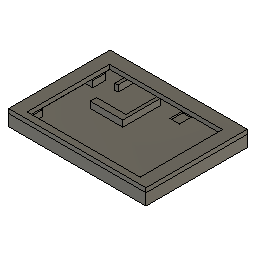
tty-buddy-enclosure (Autodesk Fusion 360 design; units mm, degrees)
part number: 2026-09-05-10-40-58-027
Autodesk Fusion 360 part; units mm, degrees
sketch "body_base" plane through (0, 0, 0) normal (0, 0, 1) x (1, 0, 0)
  line L0 (40.5, -27.25) -> (-40.5, -27.25)
  line L1 (-40.5, -27.25) -> (-40.5, 27.25)
  line L2 (-40.5, 27.25) -> (40.5, 27.25)
  line L3 (40.5, 27.25) -> (40.5, -27.25)
  line L4 (40.5, -27.25) -> (-40.5, 27.25) construction
  line L5 (-40.5, -27.25) -> (40.5, 27.25) construction
  line L6 (-40.5, 27.25) -> (40.5, 27.25)
  line L7 (40.5, 27.25) -> (40.5, 31.25)
  line L8 (40.5, 31.25) -> (-40.5, 31.25)
  line L9 (-40.5, 31.25) -> (-40.5, 27.25)
  line L10 (-43, -29.75) -> (-43, 27.25)
  line L11 (-43, 33.75) -> (-43, 27.25)
  line L12 (43, 33.75) -> (-43, 33.75)
  line L13 (43, 27.25) -> (43, 33.75)
  line L14 (43, 27.25) -> (43, -29.75)
  line L15 (43, -29.75) -> (-43, -29.75)
  circle A0 centre (-38.16, 19.88) radius 1.5
  circle A1 centre (-38.16, -19.88) radius 1.5
  circle A2 centre (38.16, -19.88) radius 1.5
  circle A3 centre (38.16, 19.88) radius 1.5
  line L16 (-25.5, 31.25) -> (-7, 31.25)
  line L17 (-7, 31.25) -> (-7, 7.75)
  line L18 (-7, 7.75) -> (-25.5, 7.75)
  line L19 (-25.5, 7.75) -> (-25.5, 31.25)
  line L20 (-40.5, -24) -> (-35.82, -24)
  line L21 (-35.82, -24) -> (-35.82, -15.76)
  line L22 (-35.82, -15.76) -> (-40.5, -15.76)
  line L23 (-40.5, -15.76) -> (-40.5, -24)
  line L24 (-40.5, -24) -> (-35.82, -15.76) construction
  line L25 (-35.82, -24) -> (-40.5, -15.76) construction
  line L26 (-40.5, 15.76) -> (-35.82, 15.76)
  line L27 (-35.82, 15.76) -> (-35.82, 24)
  line L28 (-35.82, 24) -> (-40.5, 24)
  line L29 (-40.5, 24) -> (-40.5, 15.76)
  line L30 (-40.5, 15.76) -> (-35.82, 24) construction
  line L31 (-35.82, 15.76) -> (-40.5, 24) construction
  line L32 (40.5, 24) -> (35.82, 24)
  line L33 (35.82, 24) -> (35.82, 15.76)
  line L34 (35.82, 15.76) -> (40.5, 15.76)
  line L35 (40.5, 15.76) -> (40.5, 24)
  line L36 (40.5, 24) -> (35.82, 15.76) construction
  line L37 (35.82, 24) -> (40.5, 15.76) construction
  line L38 (40.5, -15.76) -> (35.82, -15.76)
  line L39 (35.82, -15.76) -> (35.82, -24)
  line L40 (35.82, -24) -> (40.5, -24)
  line L41 (40.5, -24) -> (40.5, -15.76)
  line L42 (40.5, -15.76) -> (35.82, -24) construction
  line L43 (35.82, -15.76) -> (40.5, -24) construction
  line L44 (-7, 7.75) -> (-25.5, 7.75)
  line L45 (-25.5, 7.75) -> (-25.5, 3.75)
  line L46 (-25.5, 3.75) -> (-7, 3.75)
  line L47 (-7, 3.75) -> (-7, 7.75)
  line L48 (-7, 7.75) -> (-25.5, 3.75) construction
  line L49 (-25.5, 7.75) -> (-7, 3.75) construction
  line L50 (4.9804, -27.25) -> (19.9804, -27.25)
  line L51 (19.9804, -27.25) -> (19.9804, -22.25)
  line L52 (19.9804, -22.25) -> (4.9804, -22.25)
  line L53 (4.9804, -22.25) -> (4.9804, -27.25)
  line L54 (-25.5, 31.25) -> (-27.5, 31.25)
  line L55 (-27.5, 31.25) -> (-27.5, 21.25)
  line L56 (-27.5, 21.25) -> (-25.5, 21.25)
  line L57 (-25.5, 21.25) -> (-25.5, 31.25)
  line L58 (-7, 3.75) -> (-5, 3.75)
  line L59 (-5, 3.75) -> (-5, 27.25)
  line L60 (-5, 27.25) -> (-7, 27.25)
  line L61 (-7, 27.25) -> (-7, 3.75)
  line L62 (10.9979, 31.25) -> (4.9979, 31.25)
  line L63 (4.9979, 31.25) -> (4.9979, 23.25)
  line L64 (4.9979, 23.25) -> (10.9979, 23.25)
  line L65 (10.9979, 23.25) -> (10.9979, 31.25)
  point P0 (-38.16, 19.88)
  point P1 (-38.16, -19.88)
  point P2 (38.16, 19.88)
  point P3 (38.16, -19.88)
  point P4 (-38.16, -19.88)
  point P5 (-38.16, 19.88)
  point P6 (38.16, 19.88)
  point P7 (38.16, -19.88)
  point P8 (-16.25, 5.75)
  dimension "d1" = 81
  dimension "d2" = 54.5
  dimension "d3" = 4
  dimension "d4" = 2.5
  dimension "d13" = 3
  dimension "d14" = 3
  dimension "d15" = 3
  dimension "d16" = 3
  dimension "d20" = 18.5
  dimension "d21" = 23.5
  dimension "d24" = 8.24
  dimension "d25" = 8.24
  dimension "d29" = 18.5
  dimension "d30" = 15
  dimension "d31" = 5
  dimension "d35" = 2
  dimension "d36" = 10
  dimension "d39" = 2
  dimension "d71" = 6
  dimension "d72" = 8
  constraint horizontal L0
  constraint perpendicular L0 L1
  constraint parallel L0 L2
  constraint parallel L1 L3
  constraint coincident L4 origin
  constraint coincident L5 origin
  constraint horizontal L6
  constraint vertical L7
  constraint horizontal L8
  constraint vertical L9
  constraint coincident P5 P0
  constraint coincident P4 P1
  constraint coincident P7 P3
  constraint coincident P6 P2
  constraint horizontal L16
  constraint vertical L17
  constraint horizontal L18
  constraint vertical L19
  constraint coincident L8 L16.start
  constraint horizontal L20
  constraint perpendicular L20 L21
  constraint parallel L20 L22
  constraint parallel L21 L23
  constraint coincident L24 P4
  constraint coincident L25 P4
  constraint coincident L1 L20.start
  constraint horizontal L26
  constraint perpendicular L26 L27
  constraint parallel L26 L28
  constraint parallel L27 L29
  constraint coincident L30 P5
  constraint coincident L31 P5
  constraint horizontal L32
  constraint perpendicular L32 L33
  constraint parallel L32 L34
  constraint parallel L33 L35
  constraint coincident L36 P6
  constraint coincident L37 P6
  constraint coincident L3 L32.start
  constraint horizontal L38
  constraint perpendicular L38 L39
  constraint parallel L38 L40
  constraint parallel L39 L41
  constraint coincident L42 P7
  constraint coincident L43 P7
  constraint horizontal L44
  constraint perpendicular L44 L45
  constraint parallel L44 L46
  constraint parallel L45 L47
  constraint coincident L48 P8
  constraint coincident L49 P8
  constraint horizontal L50
  constraint vertical L51
  constraint horizontal L52
  constraint vertical L53
  constraint coincident L0 L50.start
  constraint horizontal L54
  constraint vertical L55
  constraint horizontal L56
  constraint vertical L57
  constraint horizontal L58
  constraint vertical L59
  constraint horizontal L60
  constraint vertical L61
  constraint horizontal L62
  constraint vertical L63
  constraint horizontal L64
  constraint vertical L65
  measures "d1" distance of L1.end L2.end
  measures "d2" distance of L0.end L1.end
  measures "d3" distance of L1.end L8.end
  measures "d13" diameter of A0
  measures "d14" diameter of A1
  measures "d15" diameter of A2
  measures "d16" diameter of A3
  measures "d20" distance of L16.start L16.end
  measures "d21" distance of L16.start L18.end
  measures "d24" distance of L26.end L27.end
  measures "d25" distance of L38.end L39.end
  measures "d29" distance of L45.end L46.end
  measures "d30" distance of L50.start L50.end
  measures "d31" distance of L50.start L52.end
  measures "d35" distance of L16.start L54.end
  measures "d36" distance of L16.start L56.end
  measures "d39" distance of L46.end L58.end
  measures "d71" distance of L62.start L62.end
  measures "d72" distance of L62.start L64.end
extrude "Extrude1" add sketch "body_base" against normal blind 2 contours L0 L1 L2 L3 L6 L19 L20 L21 L22 L26 L27 L28 L32 L33 L34 L38 L39 L40 L45 L46 L51 L52 L53 L55 L56 L58 L59 L63 L64 L65 | L0 L50 L51 L52 L53 | L3 L38 L39 L40 L41 | L3 L32 L33 L34 L35 | L1 L20 L21 L22 L23 | L2 L6 L7 L8 L65 | L1 L26 L27 L28 L29 | L2 L6 L63 L64 L65 | L2 L6 L8 L62 L63 L65 | L2 L6 L8 L17 L60 L63 | L2 L6 L8 L9 L55 | L2 L6 L17 L47 L58 L59 L60 L61 | L2 L6 L8 L19 L54 L55 L57 | L2 L6 L19 L55 L56 L57 | L2 L6 L17 L18 L19 L44 L57 L61 | L2 L6 L8 L16 L17 L19 L57 | L18 L44 L45 L46 L47 L61 | L10 L11 L12 L13 L14 L15 | A0 | A1 | A2 | A3 makes body 1
extrude "Extrude2" add sketch "body_base" along normal blind 3.9 contours L0 L50 L51 L52 L53 | L3 L38 L39 L40 L41 | L3 L32 L33 L34 L35 | L1 L20 L21 L22 L23 | L1 L26 L27 L28 L29 | L2 L6 L17 L47 L58 L59 L60 L61 | L2 L6 L8 L19 L54 L55 L57 | L2 L6 L19 L55 L56 L57 | L18 L44 L45 L46 L47 L61 | A0 | A1 | A2 | A3 bodies 1
extrude "Extrude3" add sketch "body_base" along normal blind 5.2 contours L10 L11 L12 L13 L14 L15 bodies 1
sketch "usb_cutout" plane through (0, 31.25, 0) normal (0, -1, 0) x (1, 0, 0)
  line L0 (-27.5, 0) -> (-27.5, 3.9)
  line L1 (-27.5, 3.9) -> (-25.5, 3.9)
  line L2 (-25.5, 0) -> (40.5, 0)
  line L3 (40.5, 0) -> (40.5, 5.2)
  line L4 (40.5, 5.2) -> (-40.5, 5.2)
  line L5 (-40.5, 5.2) -> (-40.5, 0)
  line L6 (-40.5, 0) -> (-27.5, 0)
  line L7 (-11.85, 0.7) -> (-20.65, 3.7) construction
  line L8 (-20.65, 0.7) -> (-11.85, 3.7) construction
  arc A0 (-11.55, 2.2) -> (-13.35, 4) centre (-13.35, 2.2) ccw
  line L9 (-19.15, 4) -> (-13.35, 4)
  arc A1 (-19.15, 4) -> (-20.95, 2.2) centre (-19.15, 2.2) ccw
  arc A2 (-20.95, 2.2) -> (-19.15, 0.4) centre (-19.15, 2.2) ccw
  line L10 (-13.35, 0.4) -> (-19.15, 0.4)
  arc A3 (-13.35, 0.4) -> (-11.55, 2.2) centre (-13.35, 2.2) ccw
  line L11 (-25.5, 3.9) -> (-25.5, 0)
  point P0 (-16.25, 2.2)
  dimension "d44" = 8.8
  dimension "d45" = 3
  constraint coincident L7 P0
  constraint coincident L8 P0
  measures "d44" distance of L7.end L8.end
  measures "d45" distance of L8.start L7.end
sketch "btn_cutout" plane through (0, 31.25, 0) normal (0, -1, 0) x (1, 0, 0)
  line L0 (-27.5, 0) -> (-27.5, 3.9)
  line L1 (-27.5, 3.9) -> (-25.5, 3.9)
  line L2 (-25.5, 0) -> (40.5, 0)
  line L3 (40.5, 0) -> (40.5, 5.2)
  line L4 (40.5, 5.2) -> (-40.5, 5.2)
  line L5 (-40.5, 5.2) -> (-40.5, 0)
  line L6 (-40.5, 0) -> (-27.5, 0)
  circle A0 centre (7.9979, 2) radius 1.875
  line L7 (-25.5, 3.9) -> (-25.5, 0)
  dimension "d55" = 3.75
  measures "d55" diameter of A0
extrude "Extrude4" cut sketch "usb_cutout" sketch "btn_cutout" against normal blind 2.5 contours A0 L9 A1 A2 L10 A3 of sketch 2 contours A0 bodies 1
extrude "Extrude5" cut sketch "body_base" against normal blind 1 contours L2 L6 L63 L64 L65 | L2 L6 L8 L62 L63 L65 bodies 1
sketch "lid_base" plane through (0, 0, 5.2) normal (0, 0, 1) x (-1, 0, 0)
  line L0 (40.5, -31.25) -> (-40.5, -31.25)
  line L1 (-40.5, -31.25) -> (-40.5, 27.25)
  line L2 (-40.5, 27.25) -> (40.5, 27.25)
  line L3 (40.5, 27.25) -> (40.5, -31.25)
  line L4 (-43, 29.75) -> (-43, -33.75)
  line L5 (-43, -33.75) -> (43, -33.75)
  line L6 (43, -33.75) -> (43, 29.75)
  line L7 (43, 29.75) -> (-43, 29.75)
  line L8 (43, -33.75) -> (-43, -33.75)
  line L9 (-43, -33.75) -> (-43, 29.75)
  line L10 (-43, 29.75) -> (43, 29.75)
  line L11 (43, 29.75) -> (43, -33.75)
  constraint horizontal L8
  constraint vertical L9
  constraint horizontal L10
  constraint vertical L11
  constraint coincident L4.start L7.end
  constraint coincident L5.end L6.start
extrude "Extrude6" add sketch "lid_base" along normal blind 2.7 separate body contours L0 L1 L2 L3 | L4 L5 L6 L7 L8 L9 L10 L11 makes body 2
sketch "screen_cutout" plane through (0, 0, 7.9) normal (0, 0, 1) x (-1, 0, 0)
  line L0 (43, 29.75) -> (-43, 29.75)
  line L1 (-43, 29.75) -> (-43, -33.75)
  line L2 (-43, -33.75) -> (43, -33.75)
  line L3 (43, -33.75) -> (43, 29.75)
  line L4 (40.5, -27.25) -> (-40.5, -27.25)
  line L5 (-40.5, -27.25) -> (-40.5, 27.25)
  line L6 (-40.5, 27.25) -> (40.5, 27.25)
  line L7 (40.5, 27.25) -> (40.5, -27.25)
  line L8 (-35.1, 25.5) -> (35.1, -25.5) construction
  line L9 (35.1, 25.5) -> (-35.1, -25.5) construction
  line L10 (-35.4, 25.8) -> (35.4, 25.8)
  line L11 (35.4, 25.8) -> (35.4, -25.8)
  line L12 (35.4, -25.8) -> (-35.4, -25.8)
  line L13 (-35.4, -25.8) -> (-35.4, 25.8)
  dimension "d61" = 70.2
  dimension "d62" = 51
  constraint coincident L8 origin
  constraint coincident L9 origin
  measures "d61" distance of L8.end L9.end
  measures "d62" distance of L9.start L8.end
extrude "Extrude7" cut sketch "screen_cutout" against normal blind 2.7 contours L10 L11 L12 L13 bodies 2
sketch "screw_holes" plane through (0, 0, -2) normal (0, 0, -1) x (1, 0, 0)
  line L0 (43, -33.75) -> (43, 29.75)
  line L1 (43, 29.75) -> (-43, 29.75)
  line L2 (-43, 29.75) -> (-43, -33.75)
  line L3 (-43, -33.75) -> (43, -33.75)
  circle A0 centre (38.16, -19.88) radius 1.5
  circle A1 centre (38.16, 19.88) radius 1.5
  circle A2 centre (-38.16, -19.88) radius 1.5
  circle A3 centre (-38.16, 19.88) radius 1.5
  point P0 (38.16, -19.88)
  point P1 (38.16, 19.88)
  point P2 (-38.16, -19.88)
  point P3 (-38.16, 19.88)
hole "Hole1" at (38.16, 19.88, -2) at (38.16, -19.88, -2) at (-38.16, -19.88, -2) at (-38.16, 19.88, -2) direction (0, 0, 1) diameter 2.5 depth 8.5 tip angle 180 counterbore diameter 4.3 counterbore depth 1.2 bodies 1 2
named bodies: "body", "lid"
